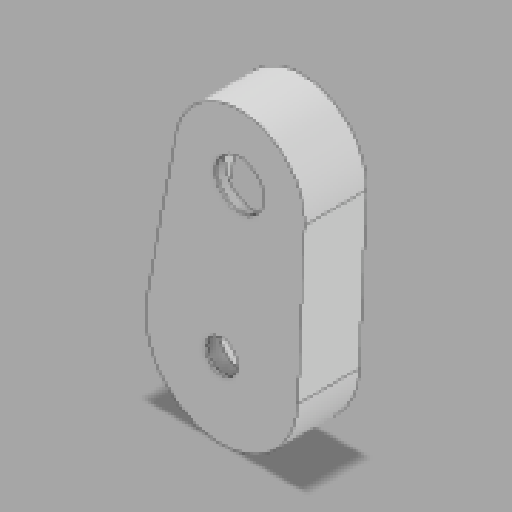
# Autodesk Inventor part: Верх редуктора
Saved by Autodesk Inventor 2025 (Build 290162000, 162)
## iProperties
Created: 2025-04-09
Part Number: Верх редуктора
Material: Типовые
Document SubType Name: Modeling
Designer: Artem Sannikov
Density: 1 g/cm^3
Appearance: По умолчанию
Author: Artem Sannikov
Autodesk Inventor part; units mm, degrees
ref_plane "YZ Plane" through (0, 0, 0) normal (1, 0, 0) x (0, 1, 0)
ref_plane "XZ Plane" through (0, 0, 0) normal (0, 1, 0) x (-1, 0, 0)
ref_plane "XY Plane" through (0, 0, 0) normal (0, 0, 1) x (1, 0, 0)
sketch "Эскиз1" plane through (0, 0, 0) normal (0, 0, 1) x (1, 0, 0)
  arc A0 (-29.2789, -52.5351) -> (18.293, -57.9783) centre (-5.684, -56.9258) ccw projected
  line L0 (18.293, -57.9783) -> (20.4803, -8.149) projected
  arc A1 (20.4803, -8.149) -> (-20.154, -3.4996) centre (0, -7.25) ccw projected
  line L1 (-20.154, -3.4996) -> (-29.2789, -52.5351) projected
  circle A2 centre (0, -7.25) radius 9.5 projected
  circle A3 centre (-5.684, -56.9258) radius 7.5 projected
  point P0 (0, 0)
extrude "Выдавливание1" add sketch "Эскиз1" against normal blind 4
sketch "Эскиз2" plane through (0, 0, -4) normal (0, 0, -1) x (-1, 0, 0)
  circle A0 centre (5.684, -56.9258) radius 7.5 projected
  circle A1 centre (5.684, -56.9258) radius 10
  point P0 (0, 0)
  dimension "d2" = 20
  constraints: 1 centre point, 1 coincident
  measures "d2" diameter of A1
extrude "Выдавливание2" add sketch "Эскиз2" along normal blind 2
sketch "Эскиз3" plane through (0, 0, 0) normal (0, 0, 1) x (1, 0, 0)
  line L0 (18.293, -57.9783) -> (20.4803, -8.149) projected
  arc A0 (20.4803, -8.149) -> (-20.154, -3.4996) centre (0, -7.25) ccw projected
  line L1 (-20.154, -3.4996) -> (-29.2789, -52.5351) projected
  arc A1 (-29.2789, -52.5351) -> (18.293, -57.9783) centre (-5.684, -56.9258) ccw projected
  circle A2 centre (-5.684, -56.9258) radius 5.1702
  circle A3 centre (0, -7.25) radius 7.692
  point P0 (0, 0)
  constraints: 2 centre point, 2 coincident
extrude "Выдавливание3" add sketch "Эскиз3" along normal blind 0.7
sketch "Эскиз4" plane through (0, 0, -4) normal (0, 0, -1) x (-1, 0, 0)
  line L0 (-20.4803, -8.149) -> (-19.6493, -27.0798) projected
  line L1 (-18.293, -57.9783) -> (-19.6493, -27.0798) projected
  arc A0 (-18.293, -57.9783) -> (29.2789, -52.5351) centre (5.684, -56.9258) ccw projected
  line L2 (23.6207, -22.1288) -> (29.2789, -52.5351) projected
  line L3 (20.154, -3.4996) -> (23.6207, -22.1288) projected
  arc A1 (20.154, -3.4996) -> (-20.4803, -8.149) centre (0, -7.25) ccw projected
  line L4 (-17.6512, -26.9921) -> (-18.4822, -8.0613)
  arc A2 (18.1878, -3.8655) -> (-18.4822, -8.0613) centre (0, -7.25) ccw
  line L5 (18.1878, -3.8655) -> (21.6544, -22.4947)
  line L6 (21.6544, -22.4947) -> (27.3127, -52.901)
  arc A3 (-16.2949, -57.8906) -> (27.3127, -52.901) centre (5.684, -56.9258) ccw
  line L7 (-16.2949, -57.8906) -> (-17.6512, -26.9921)
  point P0 (0, 0)
  dimension "d7" = 2
  constraints: 8 end point, 4 point on circle, 2 centre point, 5 other
  measures "d7" distance between parallel lines of L0 L4
ref_plane "РабПлоскость1" through (-56.4021, -90.7621, -18.8) normal (0, 0, 1) x (0.81648, -0.5773737, 0)
extrude "Выдавливание4" add sketch "Эскиз4" along normal up to surface (14.8 mm away)
sketch "Эскиз5" plane through (0, 0, 0.7) normal (0, 0, 1) x (1, 0, 0)
  arc A0 (12.2361, -11.9701) -> (12.9958, -5.4859) centre (0, -7.25) ccw projected
  arc A1 (12.2361, -11.9701) -> (15.315, -13.1578) centre (13.7756, -12.564) ccw projected
  arc A2 (16.2658, -5.042) -> (12.9958, -5.4859) centre (14.6308, -5.2639) ccw projected
  arc A3 (15.315, -13.1578) -> (16.2658, -5.042) centre (0, -7.25) ccw projected
  arc A4 (-12.2362, -2.5298) -> (-12.9958, -9.0141) centre (0, -7.25) ccw projected
  arc A5 (-12.2362, -2.5298) -> (-15.315, -1.3422) centre (-13.7756, -1.936) ccw projected
  arc A6 (-16.2658, -9.458) -> (-12.9958, -9.0141) centre (-14.6308, -9.2361) ccw projected
  arc A7 (-15.315, -1.3422) -> (-16.2658, -9.458) centre (0, -7.25) ccw projected
  point P0 (0, 0)
extrude "Выдавливание5" cut sketch "Эскиз5" against normal blind 8
